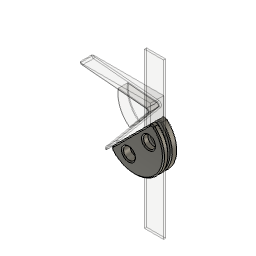
model (Autodesk Fusion 360 design; units mm, degrees)
Autodesk Fusion 360 part; units mm, degrees
sketch "Sketch1" plane through (0, 0, 0) normal (0, 1, 0) x (1, 0, 0) in component "square"
  line L0 (0, -65.75) -> (18.45, -65.75)
  line L1 (18.45, -65.75) -> (18.45, 84.25)
  line L2 (18.45, 84.25) -> (0, 84.25)
  line L3 (0, 84.25) -> (0, -65.75)
  line L4 (11.25, -28.75) -> (-57.55, -28.75)
  line L5 (-57.55, -28.75) -> (-32.65, 32.65)
  line L6 (-32.65, 32.65) -> (11.25, -11.25)
  line L7 (11.25, -11.25) -> (11.25, -28.75)
  line L8 (-56.7984, -26.8966) -> (6.2704, -21.3788)
  arc A0 (6.2704, -21.3788) -> (7.6282, -18.1008) centre (6.0961, -19.3864) ccw
  line L9 (7.6282, -18.1008) -> (-33.4016, 30.7966)
  arc A1 (-10.4518, 3.446) -> (-21.75, -23.8303) centre (6.0961, -19.3864) ccw
  dimension "d1" = 18.45
  dimension "d2" = 150
  dimension "d3" = 68.8
  dimension "d4" = 61.4
  dimension "d5" = 17.5
  dimension "d6" = 7.2
  dimension "d7" = 45
  dimension "d8" = 37
  dimension "d11" = 2
  dimension "d12" = 2
  dimension "d13" = 2
  dimension "d14" = 5
  dimension "d15" = 5
  dimension "d16" = 33
  constraint horizontal L0
  constraint vertical L1
  constraint horizontal L2
  constraint vertical L3
  constraint horizontal L4
  constraint vertical L7
  constraint coincident L3 origin
  constraint coincident L6 origin
  constraint coincident L5 L8.start
  constraint tangent L8 A0
  constraint coincident L5 L9.end
  constraint tangent A0 L9
  constraint coincident L9 A1.start
  constraint coincident L8 A1.end
  constraint coincident A0.centre A1.centre
  measures "d1" distance of L0.start L0.end
  measures "d2" distance of L0.end L1.end
  measures "d3" distance of L4.start L4.end
  measures "d4" vertical distance of L4.end L5.end
  measures "d5" distance of L4.start L6.end
  measures "d6" horizontal distance of L0.end L4.start
  measures "d7" angle of L3 L6
  measures "d8" vertical distance of L0.start L4.end
  measures "d11" distance of L4.end L8.start
  measures "d12" distance of L5.end L9.end
  measures "d13" radius of A0
  measures "d14" angle of L4 L8
  measures "d15" angle of L6 L9
  measures "d16" horizontal distance of L4.start A1.end
extrude "Extrude1" add sketch "Sketch1" along normal mid plane 2 contours L0 L1 L2 L3 L4 L6 L7 | L3 L4 L6 L7 L8 A0 L9 | L3 L8 A0 L9 makes body 1 in component "square"
extrude "Extrude2" add sketch "Sketch1" along normal mid plane 12.7 separate body contours L3 L4 L5 L8 | L3 L4 L6 L7 L8 A0 L9 | L3 L5 L6 L9 makes body 2 in component "square"
extrude "Extrude3" add sketch "Sketch1" along normal mid plane 10 separate body contours L3 L8 L9 A1 | L3 L8 A0 L9 makes body 3 in component "square"
fillet "Fillet1" radius 2 2 edges at (-56.7984, 0, 26.8966) (-33.4016, 0, -30.7966) on bodies 2 in component "square"
chamfer "Chamfer1" distance 1 angle 45 14 edges at (-24.6544, -6.35, 24.0844) (7.9439, -6.35, 20.1518) (-12.4999, -6.35, -5.8869) (-33.0715, -6.35, -30.8487) (-32.7997, -6.35, -32.2809) (-57.4042, -6.35, 28.3904) (-56.5935, -6.35, 27.1738) (-12.4999, 6.35, -5.8869) (7.9439, 6.35, 20.1518) (-24.6544, 6.35, 24.0844) (-56.5935, 6.35, 27.1738) (-57.4042, 6.35, 28.3904) (-32.7997, 6.35, -32.2809) (-33.0715, 6.35, -30.8487) on bodies 2 in component "square"
chamfer "Chamfer2" distance 0.5 angle 45 8 edges at (-7.7398, 5, 22.6045) (7.9439, 5, 20.1518) (-1.4118, 5, 7.3274) (-7.7398, -5, 22.6045) (-1.4118, -5, 7.3274) (7.9439, -5, 20.1518) (-19.9559, 5, 8.5953) (-19.9559, -5, 8.5953) on bodies 3 in component "square"
sketch "Sketch2" plane through (0, 6.35, 0) normal (0, 1, 0) x (-1, 0, 0) in component "mount"
  line L0 (56.3316, 28.4065) -> (56.4709, 28.75)
  line L1 (56.4709, 28.75) -> (-11.25, 28.75)
  line L2 (-11.25, 28.75) -> (-11.25, 11.25)
  line L3 (-11.25, 11.25) -> (31.8822, -31.8822)
  line L4 (31.8822, -31.8822) -> (32.0226, -31.5361)
  arc A0 (32.0226, -31.5361) -> (31.862, -30.5175) centre (31.0959, -31.1603) ccw
  line L5 (31.862, -30.5175) -> (-8.3943, 17.458)
  arc A1 (-6.3576, 22.375) -> (-8.3943, 17.458) centre (-6.0961, 19.3864) ccw
  line L6 (-6.3576, 22.375) -> (55.4921, 27.7861)
  arc A2 (55.4921, 27.7861) -> (56.3316, 28.4065) centre (55.4049, 28.7823) ccw
  line L7 (-18.45, -27.1913) -> (-18.45, 65.75) construction
  line L8 (0, 0) -> (0, -38.5745)
  circle A3 centre (10.1057, -24.3973) radius 2
  circle A4 centre (10.1057, -24.3973) radius 5.75
  arc A5 (0, -38.5745) -> (27.2763, -27.2763) centre (4.4439, -10.7284) ccw
  arc A6 (10.4518, -3.446) -> (21.75, 23.8303) centre (-6.0961, 19.3864) ccw construction
  line L9 (7.5861, -7.5861) -> (-15.4955, -30.6678) construction
  circle A7 centre (-9.225, -5.0666) radius 2
  circle A8 centre (-9.225, -5.0666) radius 5.75
  line L10 (-9.225, -5.0666) -> (-18.45, -5.0666) construction
  line L11 (-9.225, -5.0666) -> (0, -5.0666) construction
  arc A9 (-12.104, 12.104) -> (0, -38.5745) centre (4.4439, -10.7284) ccw
  line L12 (21.75, 23.8303) -> (10.4518, -3.446) construction
  arc A10 (10.4518, -3.446) -> (21.75, 23.8303) centre (-6.0961, 19.3864) ccw construction
  line L13 (27.2763, -27.2763) -> (0, -38.5745) construction
  line L14 (27.2763, -27.2763) -> (-12.104, 12.104) construction
  line L15 (13.6382, -32.9254) -> (0, 0) construction
  line L16 (0, 0) -> (-12.104, 12.104)
  point P0 (-18.45, 65.75)
  dimension "d25" = 4
  dimension "d26" = 11.5
  constraint vertical L7
  constraint coincident L8.start L15.end
  constraint vertical L8
  constraint coincident L3 A5.end
  constraint coincident L8 A5.start
  constraint symmetric A3 L9 A7
  constraint symmetric A4 L9 A8
  constraint coincident A7.centre A8.centre
  constraint coincident L7 L10.end
  constraint coincident L8 L11.end
  constraint horizontal L11
  constraint horizontal L10
  constraint equal L10 L11
  constraint tangent A5 A9
  constraint coincident A5.centre A9.centre
  constraint coincident L9.end A9
  constraint coincident A6.end L12.start
  constraint coincident A6.start L12.end
  constraint coincident L8.end A9
  constraint equal A5 A10
  constraint equal L12 L13
  constraint coincident L3 A9.start
  constraint midpoint L9.start L14
  constraint perpendicular L9 L14
  constraint coincident A3.centre A4.centre
  constraint coincident P0 L7.end
  constraint coincident L7.start A9
  constraint midpoint L13 L15.start
  constraint perpendicular L13 L15
  constraint coincident A3.centre L15
  measures "d25" diameter of A3
  measures "d26" diameter of A4
extrude "Extrude1'" add sketch "Sketch2" against normal up to surface (5.35 mm away) separate body contours L3 L8 A9 L16 | A4 | A8 makes body 4 at (-15.8485, 2.7833, -24.6839) makes body 5 at (2.5242, 6.35, -14.9226) in component "mount"
extrude "Extrude2'" add sketch "Sketch2" against normal up to surface (5.35 mm away) from surface at -7.35 separate body contours L3 L8 A9 L16 makes body 6 in component "mount"
extrude "Extrude3'" add sketch "Sketch2" against normal up to surface (12.7 mm away) contours L3 L8 A5 bodies 6 5 4 in component "mount"
chamfer "Chamfer1'" distance 3.75 angle 45 2 edges at (-8.241, 1, -25.1205) (11.0897, 1, -5.7898) on bodies 4 5 6 in component "mount"
fillet "Fillet1'" radius 3 3 edges at (12.104, -3.675, 12.104) (12.104, 3.675, 12.104) (-27.2763, 0, -27.2763) on bodies 6 in component "mount"
fillet "Fillet2" radius 0.5 1 edges at (0, 0, 0) on bodies 6 in component "mount"
move_face "OffsetFaces1" offset -0.2 1 faces at (12.5995, -1, 6.0725) on bodies 6 in component "mount"
chamfer "Chamfer2'" distance 1 angle 45 12 edges at (14.5859, -6.35, -2.9873) (-4.7448, -6.35, -22.318) (15.4955, -6.35, -30.6678) (-26.2523, -6.35, -27.4102) (-7.5861, -6.35, -7.5861) (12.2379, -6.35, 11.08) (22.6179, -1.2, -18.6541) (4.6745, -1.2, 4.6745) (12.2379, -1.2, 11.08) (22.6179, 1, -18.6541) (12.2379, 1, 11.08) (4.6745, 1, 4.6745) on bodies 6 in component "mount"
component "square" placed x (1, 0, 0) y (0, 1, 0) z (0, 0, 1) at (0, 0, 0)
component "mount" placed x (1, 0, 0) y (0, 1, 0) z (0, 0, 1) at (0, 0, 0)
equation "d12 = d11"
equation "d15 = d14"
equation "d17 = 1/2\""
